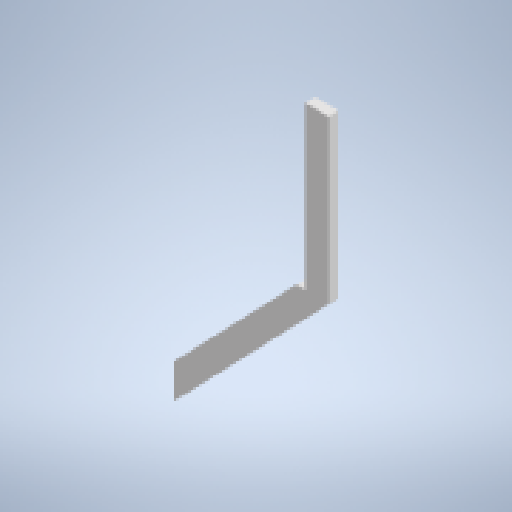
# Autodesk Inventor part: back_side
Saved by Autodesk Inventor 2025.1 (Build 291241020, 241B)
## iProperties
Created: 2024-09-20
Part Number: back_side
Material: Generic
Document SubType Name: Modeling
Designer: User
Density: 1 g/cm^3
Appearance: Default
Author: User
Autodesk Inventor part; units mm, degrees
ref_plane "YZ Plane" through (0, 0, 0) normal (1, 0, 0) x (0, 1, 0)
ref_plane "XZ Plane" through (0, 0, 0) normal (0, 1, 0) x (-1, 0, 0)
ref_plane "XY Plane" through (0, 0, 0) normal (0, 0, 1) x (1, 0, 0)
sketch "Sketch1" plane through (0, 0, 0) normal (0, 0, 1) x (1, 0, 0)
  line L0 (584.2, 1219.2) -> (673.1, 1219.2) projected
  line L1 (88.9, 0) -> (88.9, 1219.2) projected
  line L2 (584.2, 1219.2) -> (-457.2, 1219.2) projected
  line L3 (673.1, 1219.2) -> (673.1, 609.6)
  line L4 (584.2, 609.6) -> (584.2, 1219.2)
  line L5 (584.2, 1219.2) -> (673.1, 1219.2)
  line L6 (673.1, 609.6) -> (88.9, 0)
  line L7 (88.9, 0) -> (88.9, 128.4858)
  line L8 (88.9, 128.4858) -> (549.9678, 609.6)
  line L9 (549.9678, 609.6) -> (584.2, 609.6)
  point P0 (0, 0)
  constraints: 14 end point, 2 perpendicular, 1 collinear, 1 parallel, 1 point on line, 1 vertical
extrude "Extrusion1" add sketch "Sketch1" against normal blind 38.1 contours L0 L3 L6 L1 L8 L9 L4
body "Solid1"
